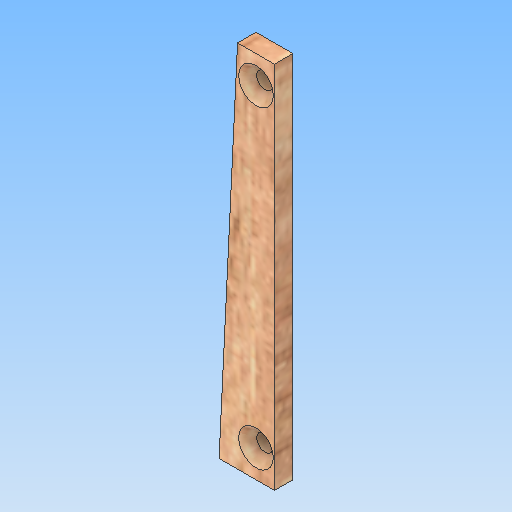
# Autodesk Inventor part: Pancake_Side Piece
Saved by Autodesk Inventor 2018.1 (Build 221171000, 171)
## iProperties
Created: 2019-02-21
Part Number: Pancake_Side Piece
Material: Wood (Birch)
Document SubType Name: Modeling
Designer: James
Density: 0.55 g/cm^3
Appearance: Birch - Natural Polished
Mass: 3.28641 g
Surface Area: 36.7842 cm^2
Volume: 5.9753 cm^3
Author: James
Autodesk Inventor part; units mm, degrees
ref_plane "YZ Plane" through (0, 0, 0) normal (1, 0, 0) x (0, 1, 0)
ref_plane "XZ Plane" through (0, 0, 0) normal (0, 1, 0) x (-1, 0, 0)
ref_plane "XY Plane" through (0, 0, 0) normal (0, 0, 1) x (1, 0, 0)
sketch "Sketch1" plane through (0, 0, 0) normal (0, 0, 1) x (1, 0, 0)
  line L0 (0, 0) -> (-15, 0)
  line L1 (-10, 100) -> (0, 100)
  line L2 (0, 100) -> (0, 0)
  line L3 (-15, 0) -> (-10, 100)
  dimension "d0" = 5
  dimension "d1" = 100
  dimension "d2" = 15
  constraints: 8 end point, 1 horizontal, 1 parallel, 1 vertical
  measures "d0" horizontal distance of L1.start L0.end
  measures "d1" distance of L1.end L0.start
  measures "d2" distance of L0.start L0.end
extrude "Extrusion1" add sketch "Sketch1" along normal blind 5
sketch "Sketch2" plane through (0, 0, 5) normal (0, 0, 1) x (1, 0, 0)
  line L0 (0, 100) -> (-10, 100) projected
  line L1 (0, 0) -> (0, 100) projected
  line L2 (-15, 0) -> (0, 0) projected
  point P0 (-5, 92.5)
  point P1 (-5, 7.5)
  dimension "d5" = 7.5
  dimension "d6" = 5
  dimension "d7" = 7.5
  constraints: 1 vertical alignment
  measures "d5" distance from line of point (-5, 92.5) L0
  measures "d6" distance from line of L1 point (-5, 92.5)
  measures "d7" distance from line of L2 point (-5, 7.5)
hole "Hole1" at (-5, 92.5, 5) at (-5, 7.5, 5) direction (0, 0, -1) diameter 4.5 end through all countersink diameter 9.4 countersink angle 90 clearance for "Flat Head Machine Screw" size "M4" standard "Ansi Metric M Profile"
equation "\"d7\" = d5"
body "Solid1"
